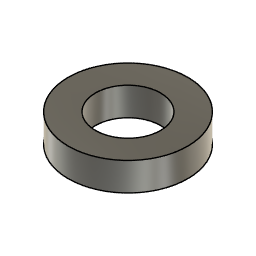
Fermoire_bouteille (Autodesk Fusion 360 archive; units mm, degrees)
design "roulement"
Autodesk Fusion 360 part; units mm, degrees
sketch "Esquisse1" plane through (0, 0, 0) normal (0, 0, 1) x (1, 0, 0)
  circle A0 centre (0, 0) radius 27.525
  circle A1 centre (0, 0) radius 15
  dimension "d1" = 55.05
  dimension "d2" = 30
  constraint coincident A0.centre A1.centre
  measures "d1" diameter of A0
  measures "d2" diameter of A1
extrude "Extrusion1" add sketch "Esquisse1" along normal blind 13
